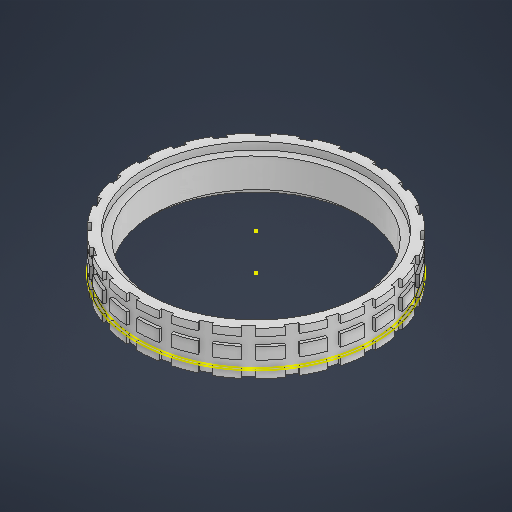
# Autodesk Inventor part: Ruedas_Rover
Saved by Autodesk Inventor 2026 (Build 300175000, 175)
## iProperties
Created: 2025-09-04
Part Number: Ruedas_Rover
Material: Generic
Document SubType Name: Modeling
Designer: Nicolás De Bruijn
Density: 1 g/cm^3
Appearance: Default
Author: Nicolás De Bruijn
Autodesk Inventor part; units mm, degrees
ref_plane "YZ Plane" through (0, 0, 0) normal (1, 0, 0) x (0, 1, 0)
ref_plane "XZ Plane" through (0, 0, 0) normal (0, 1, 0) x (-1, 0, 0)
sketch "Sketch1" plane through (0, 0, 0) normal (0, 1, 0) x (-1, 0, 0)
  arc A0 (-2, -1.5) -> (-2, 1.5) centre (0, 0) ccw
  line L0 (-2, 1.5) -> (-2, -1.5)
  circle A1 centre (0, 0) radius 7.5
  circle A2 centre (0, 0) radius 37.5
  circle A3 centre (0, 0) radius 40
  line L1 (0, -7.5) -> (0, -37.5)
  line L2 (5.3033, -5.3033) -> (26.5165, -26.5165)
  line L3 (7.5, 0) -> (37.5, 0)
  line L4 (5.3033, 5.3033) -> (26.5165, 26.5165)
  line L5 (0, 7.5) -> (0, 37.5)
  line L6 (-5.3033, 5.3033) -> (-26.5165, 26.5165)
  line L7 (-7.5, 0) -> (-37.5, 0)
  line L8 (-5.3033, -5.3033) -> (-26.5165, -26.5165)
  point P0 (-7.5, 0)
  point P1 (0, 37.5)
  point P2 (5.3033, 5.3033)
  point P3 (37.5, 0)
  dimension "d2" = 15
  dimension "d0" = 5
  dimension "d1" = 2
  dimension "d11" = 360
  dimension "d15" = 2.5
  dimension "d16" = 80
  constraints: 18 end point, 3 coincident, 2 centre point, 2 point on circle, 2 vertical, 31 other
  measures "d0" diameter of A0
  measures "d1" distance from line of L0 point (0, 0)
  measures "d16" diameter of A3
extrude "Extrusion1" add sketch "Sketch1" along normal blind 10 contours A1 | L3 A2 L2 A1 | A1 L5 A2 L4 | L1 A2 L8 A1 | A1 L7 A2 L6 | A3
sketch "Sketch3" plane through (0, 0, 0) normal (0, -1, 0) x (1, 0, 0)
  circle A0 centre (0, 0) radius 40 projected
  arc A1 (2, 1.5) -> (2, -1.5) centre (0, 0) ccw projected
  circle A2 centre (0, 0) radius 37.5
  constraints: 1 centre point, 1 coincident
extrude "Extrusion2" add sketch "Sketch3" along normal blind 5
sketch "Sketch4" plane through (0, 10, 0) normal (0, 1, 0) x (1, 0, 0)
  point P0 (0, 0)
sketch "Sketch5" plane through (0, 10, 0) normal (0, 1, 0) x (1, 0, 0)
  circle A0 centre (0, 0) radius 41
  circle A1 centre (0, 0) radius 40 projected
  dimension "d17" = 82
  constraints: 1 centre point, 1 coincident
  measures "d17" diameter of A0
extrude "Extrusion3" add sketch "Sketch5" against normal blind 2.5
sketch "Sketch6" plane through (0, -5, 0) normal (0, -1, 0) x (1, 0, 0)
  circle A0 centre (0, 0) radius 41 projected
  circle A1 centre (0, 0) radius 40 projected
extrude "Extrusion4" add sketch "Sketch6" against normal blind 2.5
sketch "Sketch7" plane through (0, -2.5, 0) normal (0, 1, 0) x (1, 0, 0)
  circle A0 centre (0, 0) radius 40 projected
  circle A1 centre (0, 0) radius 41 projected
ref_plane "Work Plane1" through (0, 2.5, 0) normal (0, 1, 0) x (1, 0, 0)
sketch "Sketch8" plane through (0, 2.5, 0) normal (0, 1, 0) x (1, 0, 0)
  circle A0 centre (0, 0) radius 40 projected
  circle A1 centre (0, 0) radius 41 projected
extrude "Extrusion5" add sketch "Sketch8" along normal blind 2 and the other way blind 2
sketch "Sketch9" plane through (0, 10, 0) normal (0, 1, 0) x (1, 0, 0)
  circle A0 centre (0, 0) radius 40 projected
  circle A1 centre (0, 0) radius 41 projected
  line L0 (0, 40) -> (0, 41)
  line L1 (3.4862, 39.8478) -> (3.5734, 40.844)
  line L2 (0, 0) -> (41, 0) construction
  line L3 (-10.3528, 38.637) -> (-10.6116, 39.603)
  line L4 (-6.9459, 39.3923) -> (-7.1196, 40.3771)
  line L5 (-20, 34.641) -> (-20.5, 35.507)
  line L6 (-16.9047, 36.2523) -> (-17.3273, 37.1586)
  line L7 (-28.2843, 28.2843) -> (-28.9914, 28.9914)
  line L8 (-25.7115, 30.6418) -> (-26.3543, 31.4078)
  line L9 (-34.641, 20) -> (-35.507, 20.5)
  line L10 (-32.7661, 22.9431) -> (-33.5852, 23.5166)
  line L11 (-38.637, 10.3528) -> (-39.603, 10.6116)
  line L12 (-37.5877, 13.6808) -> (-38.5274, 14.0228)
  line L13 (-40, 0) -> (-41, 0)
  line L14 (-39.8478, 3.4862) -> (-40.844, 3.5734)
  line L15 (-38.637, -10.3528) -> (-39.603, -10.6116)
  line L16 (-39.3923, -6.9459) -> (-40.3771, -7.1196)
  line L17 (-34.641, -20) -> (-35.507, -20.5)
  line L18 (-36.2523, -16.9047) -> (-37.1586, -17.3273)
  line L19 (-28.2843, -28.2843) -> (-28.9914, -28.9914)
  line L20 (-30.6418, -25.7115) -> (-31.4078, -26.3543)
  line L21 (-20, -34.641) -> (-20.5, -35.507)
  line L22 (-22.9431, -32.7661) -> (-23.5166, -33.5852)
  line L23 (-10.3528, -38.637) -> (-10.6116, -39.603)
  line L24 (-13.6808, -37.5877) -> (-14.0228, -38.5274)
  line L25 (0, -40) -> (0, -41)
  line L26 (-3.4862, -39.8478) -> (-3.5734, -40.844)
  line L27 (10.3528, -38.637) -> (10.6116, -39.603)
  line L28 (6.9459, -39.3923) -> (7.1196, -40.3771)
  line L29 (20, -34.641) -> (20.5, -35.507)
  line L30 (16.9047, -36.2523) -> (17.3273, -37.1586)
  line L31 (28.2843, -28.2843) -> (28.9914, -28.9914)
  line L32 (25.7115, -30.6418) -> (26.3543, -31.4078)
  line L33 (34.641, -20) -> (35.507, -20.5)
  line L34 (32.7661, -22.9431) -> (33.5852, -23.5166)
  line L35 (38.637, -10.3528) -> (39.603, -10.6116)
  line L36 (37.5877, -13.6808) -> (38.5274, -14.0228)
  line L37 (40, 0) -> (41, 0)
  line L38 (39.8478, -3.4862) -> (40.844, -3.5734)
  line L39 (38.637, 10.3528) -> (39.603, 10.6116)
  line L40 (39.3923, 6.9459) -> (40.3771, 7.1196)
  line L41 (34.641, 20) -> (35.507, 20.5)
  line L42 (36.2523, 16.9047) -> (37.1586, 17.3273)
  line L43 (28.2843, 28.2843) -> (28.9914, 28.9914)
  line L44 (30.6418, 25.7115) -> (31.4078, 26.3543)
  line L45 (20, 34.641) -> (20.5, 35.507)
  line L46 (22.9431, 32.7661) -> (23.5166, 33.5852)
  line L47 (10.3528, 38.637) -> (10.6116, 39.603)
  line L48 (13.6808, 37.5877) -> (14.0228, 38.5274)
  point P0 (40, 0)
  dimension "d33" = 360
  constraints: 98 end point, 1 horizontal, 1 vertical, 150 other
extrude "Extrusion7" cut sketch "Sketch9" against normal through all contours L37 A1 L38 A0 | A0 L39 A1 L40 | L35 A1 L36 A0 | A0 L41 A1 L42 | L33 A1 L34 A0 | A0 L43 A1 L44 | L31 A1 L32 A0 | A0 L45 A1 L46 | L29 A1 L30 A0 | A0 L47 A1 L48 | L27 A1 L28 A0 | A0 L0 A1 L1 | L25 A1 L26 A0 | A0 L3 A1 L4 | L23 A1 L24 A0 | A0 L5 A1 L6 | L21 A1 L22 A0 | A0 L7 A1 L8 | L19 A1 L20 A0 | A0 L9 A1 L10 | L17 A1 L18 A0 | A0 L11 A1 L12 | L15 A1 L16 A0 | A0 L13 A1 L14
sketch "Sketch10" plane through (0, 10, 0) normal (0, 1, 0) x (1, 0, 0)
  line L0 (-37.5, 0) -> (-7.5, 0) projected
  line L1 (-5.3033, 5.3033) -> (-26.5165, 26.5165) projected
  line L2 (-12.0711, 5) -> (-26.6742, 19.6031)
  line L3 (-12.0711, 5) -> (-32.723, 5)
  line L4 (-32.723, 5) -> (-26.6742, 19.6031)
  line L5 (-5, -12.0711) -> (-19.6031, -26.6742)
  line L6 (-5, -32.723) -> (-19.6031, -26.6742)
  line L7 (-5, -12.0711) -> (-5, -32.723)
  line L8 (12.0711, -5) -> (26.6742, -19.6031)
  line L9 (32.723, -5) -> (26.6742, -19.6031)
  line L10 (12.0711, -5) -> (32.723, -5)
  line L11 (5, 12.0711) -> (19.6031, 26.6742)
  line L12 (5, 32.723) -> (19.6031, 26.6742)
  line L13 (5, 12.0711) -> (5, 32.723)
  point P0 (0, 0)
  dimension "d37" = 5
  dimension "d38" = 5
  dimension "d42" = 360
  constraints: 24 end point, 2 parallel, 25 other
  measures "d37" distance between parallel lines of L1 L2
  measures "d38" distance between parallel lines of L0 L3
extrude "Extrusion8" cut sketch "Sketch10" against normal through all
sketch "Sketch11" plane through (0, 10, 0) normal (0, 1, 0) x (1, 0, 0)
  arc A0 (-37.5, 0) -> (-26.5165, -26.5165) centre (0, 0) ccw projected
  circle A1 centre (0, 0) radius 37.5
  point P0 (-26.5165, -26.5165)
  constraints: 1 centre point, 1 coincident
extrude "Extrusion9" cut sketch "Sketch11" against normal through all
sketch "Sketch13" plane through (0, -5, 0) normal (0, -1, 0) x (1, 0, 0)
  circle A0 centre (0, 0) radius 37.5 projected
  circle A1 centre (0, 0) radius 35
  circle A2 centre (0, 0) radius 37.5
  dimension "d48" = 70
  constraints: 2 centre point, 2 coincident, 1 concentric
  measures "d48" diameter of A1
extrude "Extrusion10" add sketch "Sketch13" against normal blind 15
sketch "Sketch14" plane through (0, 10, 0) normal (0, 1, 0) x (1, 0, 0)
  circle A0 centre (0, 0) radius 35 projected
  circle A1 centre (0, 0) radius 37.5
  dimension "d51" = 75
  constraints: 1 centre point, 1 coincident
  measures "d51" diameter of A1
extrude "Extrusion11" cut sketch "Sketch14" against normal blind 2.5
sketch "Sketch15" plane through (0, -5, 0) normal (0, -1, 0) x (1, 0, 0)
  circle A0 centre (0, 0) radius 37.5
  circle A1 centre (0, 0) radius 35 projected
  dimension "d54" = 75
  constraints: 1 centre point, 1 coincident
  measures "d54" diameter of A0
extrude "Extrusion12" cut sketch "Sketch15" against normal blind 2.5
body "Solid1"
